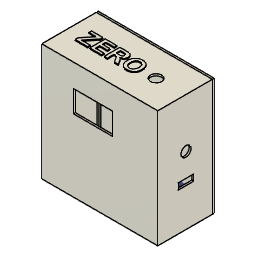
DigitalAngleGauge (Autodesk Fusion 360 design; units mm, degrees)
Autodesk Fusion 360 part; units mm, degrees
note: some values were not read from the file. Set by a fixed rule: which face or edge a step refers to.
sketch "Sketch1" plane through (0, 0, 0) normal (0, 1, 0) x (1, 0, 0)
  line L0 (0, 0) -> (74.4, 0)
  line L1 (74.4, 0) -> (74.4, -35)
  line L2 (74.4, -35) -> (0, -35)
  line L3 (0, -35) -> (0, 0)
  dimension "d15" = 74.4
  dimension "d16" = 35
  constraint horizontal L0
  constraint vertical L1
  constraint horizontal L2
  constraint vertical L3
  constraint coincident L0.start L3.end
  measures "d15" distance of L0.start L0.end
  measures "d16" distance of L0.start L2.end
extrude "Extrude1" add sketch "Sketch1" along normal blind 75 makes body 1
sketch "Sketch2" plane through (0, 0, 0) normal (0, -1, 0) x (1, 0, 0)
  line L0 (74.4, 35) -> (0, 35)
  line L1 (0, 35) -> (0, 0)
  line L2 (0, 0) -> (74.4, 0)
  line L3 (74.4, 0) -> (74.4, 35)
  line L4 (37.2, 0) -> (37.2, 35) construction
  line L5 (0, 35) -> (37.2, 0) construction
  line L6 (37.2, 0) -> (74.4, 35) construction
  circle A0 centre (18.6, 17.5) radius 4.2
  circle A1 centre (55.8, 17.5) radius 4.2
  dimension "d20" = 8.4
  dimension "d21" = 8.4
  constraint midpoint L2 L4.start
  constraint midpoint L0 L4.end
  constraint coincident L0.end L1.start
  constraint coincident L0.start L3.end
  constraint midpoint L5 A0.centre
  constraint midpoint L6 A1.centre
  measures "d20" diameter of A0
  measures "d21" diameter of A1
extrude "Extrude2" cut sketch "Sketch2" against normal blind 2.2 contours A0 | A1 bodies 1
shell "Shell1" thickness 1.2 removed faces 1 at (24.8, 25, 0) on bodies 1
sketch "Sketch3" plane through (0, 75, 0) normal (0, 1, 0) x (-1, 0, 0)
  line L0 (0, 35) -> (-74.4, 35)
  line L1 (-74.4, 35) -> (-74.4, 0)
  line L2 (-74.4, 0) -> (0, 0)
  line L3 (0, 0) -> (0, 35)
  line L4 (-37.2, 35) -> (-74.4, 0) construction
  circle A0 centre (-55.8, 17.5) radius 3.6
  dimension "d29" = 7.2
  constraint midpoint L0 L4.start
  constraint coincident L1.end L2.start
  constraint midpoint L4 A0.centre
  measures "d29" diameter of A0
extrude "Extrude3" cut sketch "Sketch3" against normal up to surface (1.2 mm away) contours A0 bodies 1
sketch "Sketch4" plane through (0, 75, 0) normal (0, 1, 0) x (-1, 0, 0)
  circle A0 centre (-55.8, 17.5) radius 3.6
  line L0 (0, 35) -> (-74.4, 35)
  line L1 (-74.4, 35) -> (-74.4, 0)
  line L2 (-74.4, 0) -> (0, 0)
  line L3 (0, 0) -> (0, 35)
  line L4 (0, 35) -> (-55.8, 35) construction
  line L5 (-55.8, 35) -> (-55.8, 0) construction
  line L6 (-55.8, 0) -> (0, 0) construction
  line L7 (0, 0) -> (0, 35) construction
  dimension "d32" = 10
  text T0 "ZERO" font "Arial" height 10 bold align centre middle in box 55.8 x 35 at (0, 35) x (-1, 0) y (0, -1) spacing 1 kerned
  constraint coincident L0
  constraint coincident L2.end
  constraint coincident A0.centre L5
extrude "Extrude4" add sketch "Sketch4" along normal blind 0.6 text T0 bodies 1
sketch "Sketch5" plane through (1.2, 0, 0) normal (1, 0, 0) x (0, 0, -1)
  line L0 (-33.8, 1.2) -> (0, 1.2)
  line L1 (0, 1.2) -> (0, 73.8)
  line L2 (0, 73.8) -> (-33.8, 73.8)
  line L3 (-33.8, 73.8) -> (-33.8, 1.2)
  line L4 (-33.8, 12.4) -> (0, 12.4) construction
  line L5 (-12.1, 3.4) -> (-22.9, 3.4) construction
  circle A0 centre (-16.9, 12.4) radius 9
  dimension "d36" = 9
  dimension "d37" = 18
  constraint coincident L3 L4.start
  constraint coincident L1 L4.end
  constraint perpendicular L3 L4
  constraint midpoint L4 A0.centre
  measures "d36" distance of L4 L5
  measures "d37" diameter of A0
extrude "Extrude5" add sketch "Sketch5" along normal up to surface (72 mm away) separate body contours A0 makes body 2
sketch "Sketch6" plane through (1.2, 0, 0) normal (1, 0, 0) x (0, 0, -1)
  line L0 (-33.8, 1.2) -> (0, 1.2)
  line L1 (0, 1.2) -> (0, 73.8)
  line L2 (0, 73.8) -> (-33.8, 73.8)
  line L3 (-33.8, 73.8) -> (-33.8, 1.2)
  line L4 (-27.6, 67.1397) -> (-6.2, 67.1397) construction
  line L5 (-6.2, 67.1397) -> (-6.2, 23.6397) construction
  line L6 (-6.2, 23.6397) -> (-27.6, 23.6397) construction
  line L7 (-27.6, 23.6397) -> (-27.6, 67.1397) construction
  line L8 (-6.2, 67.1397) -> (0, 67.1397) construction
  line L9 (-27.6, 67.1397) -> (-33.8, 67.1397) construction
  circle A0 centre (-9.2, 61) radius 1.2
  circle A1 centre (-25.2, 31) radius 1.2
  dimension "d40" = 21.4
  dimension "d41" = 43.5
  dimension "d42" = 3
  dimension "d43" = 19
  dimension "d44" = 2.4
  dimension "d45" = 2.4
  constraint horizontal L4
  constraint vertical L5
  constraint horizontal L6
  constraint vertical L7
  constraint coincident L1 L8.end
  constraint perpendicular L1 L8
  constraint coincident L3 L9.end
  constraint perpendicular L3 L9
  constraint equal L8 L9
  measures "d40" distance of L4.start L4.end
  measures "d41" distance of L4.start L6.end
  measures "d42" distance of L5 A0.centre
  measures "d43" distance of L5 A1.centre
  measures "d44" diameter of A1
  measures "d45" diameter of A0
extrude "Extrude6" add sketch "Sketch6" along normal blind 4 contours A0 | A1 bodies 1
sketch "Sketch7" plane through (73.2, 0, 0) normal (-1, 0, 0) x (0, 0, 1)
  line L0 (0, 1.2) -> (33.8, 1.2)
  line L1 (33.8, 1.2) -> (33.8, 73.8)
  line L2 (33.8, 73.8) -> (0, 73.8)
  line L3 (0, 73.8) -> (0, 1.2)
  line L4 (7.9, 24.4) -> (25.9, 24.4) construction
  line L5 (25.9, 24.4) -> (25.9, 22.4) construction
  line L6 (25.9, 22.4) -> (7.9, 22.4) construction
  line L7 (7.9, 22.4) -> (7.9, 24.4) construction
  line L8 (7.9, 24.4) -> (0, 24.4) construction
  line L9 (25.9, 24.4) -> (33.8, 24.4) construction
  circle A0 centre (16.9, 12.4) radius 9 construction
  line L10 (11.9, 24.4) -> (21.9, 24.4)
  line L11 (21.9, 24.4) -> (21.9, 28.4)
  line L12 (21.9, 28.4) -> (11.9, 28.4)
  line L13 (11.9, 28.4) -> (11.9, 24.4)
  line L14 (21.9, 28.4) -> (25.9, 24.4) construction
  line L15 (11.9, 28.4) -> (7.9, 24.4) construction
  dimension "d48" = 2
  dimension "d49" = 18
  dimension "d50" = 10
  dimension "d51" = 10
  dimension "d52" = 4
  constraint horizontal L4
  constraint vertical L5
  constraint horizontal L6
  constraint vertical L7
  constraint coincident L3 L8.end
  constraint perpendicular L3 L8
  constraint coincident L1 L9.end
  constraint perpendicular L1 L9
  constraint equal L8 L9
  constraint horizontal L10
  constraint vertical L11
  constraint horizontal L12
  constraint vertical L13
  constraint coincident L4 L10.start
  constraint equal L14 L15
  measures "d48" distance of L4.start L6.end
  measures "d49" distance of L4.start L4.end
  measures "d50" distance of L6 A0.centre
  measures "d51" distance of L11.end L12.end
  measures "d52" distance of L10.end L11.end
extrude "Extrude7" cut sketch "Sketch7" against normal up to surface (1.2 mm away) contours L10 L11 L12 L13 bodies 1
sketch "Sketch8" plane through (73.2, 0, 0) normal (-1, 0, 0) x (0, 0, 1)
  line L0 (11.9, 28.4) -> (21.9, 28.4)
  line L1 (21.9, 28.4) -> (21.9, 24.4)
  line L2 (21.9, 24.4) -> (11.9, 24.4)
  line L3 (11.9, 24.4) -> (11.9, 28.4)
  line L4 (0, 1.2) -> (33.8, 1.2)
  line L5 (33.8, 1.2) -> (33.8, 73.8)
  line L6 (33.8, 73.8) -> (0, 73.8)
  line L7 (0, 73.8) -> (0, 1.2)
  circle A0 centre (16.9, 43.4) radius 3.25
  line L8 (16.9, 43.4) -> (0, 43.4) construction
  line L9 (16.9, 43.4) -> (33.8, 43.4) construction
  dimension "d55" = 15
  dimension "d56" = 6.5
  constraint coincident A0.centre L8.start
  constraint coincident L7 L8.end
  constraint perpendicular L7 L8
  constraint coincident L5 L9.end
  constraint perpendicular L5 L9
  constraint equal L8 L9
  measures "d55" distance of L0 A0.centre
  measures "d56" diameter of A0
extrude "Extrude8" cut sketch "Sketch8" against normal up to surface (1.2 mm away) contours A0 bodies 1
sketch "Sketch9" plane through (0, 0, 33.8) normal (0, 0, -1) x (-1, 0, 0)
  line L0 (-73.2, 1.2) -> (-1.2, 1.2)
  line L1 (-1.2, 1.2) -> (-1.2, 73.8)
  line L2 (-1.2, 73.8) -> (-73.2, 73.8)
  line L3 (-73.2, 73.8) -> (-73.2, 1.2)
  line L4 (-1.2, 68.2) -> (-14.2, 68.2) construction
  line L5 (-14.2, 68.2) -> (-14.2, 25.2) construction
  line L6 (-14.2, 25.2) -> (-1.2, 25.2) construction
  line L7 (-1.2, 25.2) -> (-1.2, 68.2) construction
  line L8 (-5.2, 62.2) -> (-5.2, 59.8) construction
  line L9 (-1.2, 59.8) -> (-1.2, 62.2) construction
  line L10 (-73.2, 73.8) -> (-50.2, 73.8) construction
  line L11 (-50.2, 73.8) -> (-50.2, 21.4) construction
  line L12 (-50.2, 21.4) -> (-73.2, 21.4) construction
  line L13 (-73.2, 21.4) -> (-73.2, 73.8) construction
  line L14 (-1.2, 21.4) -> (-1.2, 3.4) construction
  line L15 (-73.2, 21.4) -> (-73.2, 3.4) construction
  line L16 (-46.4, 65.8) -> (-19.2, 65.8) construction
  line L17 (-19.2, 65.8) -> (-19.2, 37.8) construction
  line L18 (-19.2, 37.8) -> (-46.4, 37.8) construction
  line L19 (-46.4, 37.8) -> (-46.4, 65.8) construction
  line L20 (-45.3, 60.3) -> (-20.3, 60.3)
  line L21 (-20.3, 60.3) -> (-20.3, 46.3)
  line L22 (-20.3, 46.3) -> (-45.3, 46.3)
  line L23 (-45.3, 46.3) -> (-45.3, 60.3)
  line L24 (-45.3, 53.3) -> (-46.4, 53.3) construction
  line L25 (-20.3, 53.3) -> (-19.2, 53.3) construction
  line L26 (-46.4, 37.8) -> (-42.6, 37.8)
  line L27 (-42.6, 37.8) -> (-42.6, 36.6)
  line L28 (-42.6, 36.6) -> (-47.6, 36.6)
  line L29 (-47.6, 36.6) -> (-47.6, 41.6)
  line L30 (-47.6, 41.6) -> (-46.4, 41.6)
  line L31 (-46.4, 37.8) -> (-46.4, 41.6)
  line L32 (-46.4, 37.8) -> (-19.2, 65.8) construction
  line L33 (-19.2, 37.8) -> (-46.4, 65.8) construction
  line L34 (-19.2, 37.8) -> (-23, 37.8)
  line L35 (-23, 37.8) -> (-23, 36.6)
  line L36 (-23, 36.6) -> (-18, 36.6)
  line L37 (-18, 36.6) -> (-18, 41.6)
  line L38 (-18, 41.6) -> (-19.2, 41.6)
  line L39 (-19.2, 37.8) -> (-19.2, 41.6)
  line L40 (-19.2, 62) -> (-18, 62)
  line L41 (-18, 62) -> (-18, 67)
  line L42 (-18, 67) -> (-23, 67)
  line L43 (-23, 67) -> (-23, 65.8)
  line L44 (-19.2, 65.8) -> (-23, 65.8)
  line L45 (-19.2, 65.8) -> (-19.2, 62)
  line L46 (-46.4, 65.8) -> (-42.6, 65.8)
  line L47 (-42.6, 65.8) -> (-42.6, 67)
  line L48 (-42.6, 67) -> (-47.6, 67)
  line L49 (-47.6, 67) -> (-47.6, 62)
  line L50 (-47.6, 62) -> (-46.4, 62)
  line L51 (-46.4, 65.8) -> (-46.4, 62)
  dimension "d59" = 13
  dimension "d60" = 43
  dimension "d61" = 6
  dimension "d62" = 23
  dimension "d63" = 27.2
  dimension "d64" = 28
  dimension "d65" = 5
  dimension "d66" = 8
  dimension "d67" = 5.5
  dimension "d68" = 25
  dimension "d69" = 14
  dimension "d70" = 1.2
  dimension "d71" = 1.2
  dimension "d72" = 5
  dimension "d73" = 5
  dimension "d74" = 1.2
  dimension "d75" = 1.2
  dimension "d76" = 1.2
  dimension "d77" = 1.2
  dimension "d78" = 5
  dimension "d79" = 5
  dimension "d80" = 5
  dimension "d81" = 5
  dimension "d82" = 1.2
  dimension "d83" = 1.2
  dimension "d84" = 5
  dimension "d85" = 5
  constraint horizontal L4
  constraint vertical L5
  constraint horizontal L6
  constraint vertical L7
  constraint coincident L1 L4.start
  constraint horizontal L10
  constraint vertical L11
  constraint horizontal L12
  constraint vertical L13
  constraint coincident L3 L2.end
  constraint collinear L2 L10
  constraint coincident L12 L13.start
  constraint horizontal L16
  constraint vertical L17
  constraint horizontal L18
  constraint vertical L19
  constraint horizontal L20
  constraint vertical L21
  constraint horizontal L22
  constraint vertical L23
  constraint midpoint L23 L24.start
  constraint coincident L19 L24.end
  constraint perpendicular L19 L24
  constraint midpoint L21 L25.start
  constraint coincident L17 L25.end
  constraint perpendicular L17 L25
  constraint equal L24 L25
  constraint coincident L18 L26.end
  constraint perpendicular L19 L26
  constraint perpendicular L26 L27
  constraint perpendicular L27 L28
  constraint perpendicular L28 L29
  constraint coincident L19 L30.end
  constraint perpendicular L19 L30
  constraint coincident L18 L34.end
  constraint perpendicular L17 L34
  constraint perpendicular L18 L35
  constraint perpendicular L35 L36
  constraint perpendicular L36 L37
  constraint coincident L17 L38.end
  constraint perpendicular L17 L38
  constraint coincident L17 L40.start
  constraint perpendicular L17 L40
  constraint perpendicular L40 L41
  constraint perpendicular L17 L42
  constraint coincident L16 L43.end
  constraint perpendicular L16 L43
  constraint coincident L16 L46.end
  constraint perpendicular L19 L46
  constraint perpendicular L46 L47
  constraint perpendicular L47 L48
  constraint perpendicular L46 L49
  constraint coincident L19 L50.end
  constraint perpendicular L19 L50
  measures "d59" distance of L4.start L4.end
  measures "d60" distance of L4.end L5.end
  measures "d61" distance of L4 L8.start
  measures "d62" distance of L2.end L10.end
  measures "d63" distance of L16.start L16.end
  measures "d64" distance of L16.start L18.end
  measures "d65" distance of L5 L17
  measures "d66" distance of L2 L16
  measures "d67" distance of L16 L20
  measures "d68" distance of L20.start L20.end
  measures "d69" distance of L20.start L22.end
  measures "d70" distance of L18 L28
  measures "d71" distance of L19 L29
  measures "d72" distance of L28 L30
  measures "d73" distance of L27 L29
  measures "d74" distance of L40.start L40.end
  measures "d75" distance of L42.end L43.end
  measures "d76" distance of L37.end L38.end
  measures "d77" distance of L34.end L35.end
  measures "d78" distance of L35.end L36.end
  measures "d79" distance of L36.end L37.end
  measures "d80" distance of L40.end L41.end
  measures "d81" distance of L41.end L42.end
  measures "d82" distance of L49.end L50.end
  measures "d83" distance of L46.end L47.end
  measures "d84" distance of L47.end L48.end
  measures "d85" distance of L48.end L49.end
extrude "Extrude9" cut sketch "Sketch9" against normal up to surface (1.2 mm away) contours L20 L21 L22 L23 bodies 1
extrude "Extrude10" add sketch "Sketch9" along normal blind 4 contours L26 L27 L28 L29 L30 L31 | L34 L35 L36 L37 L38 L39 | L40 L41 L42 L43 L44 L45 | L46 L47 L48 L49 L50 L51 bodies 1
sketch "Sketch10" plane through (0, 0, 0) normal (0, 0, -1) x (-1, 0, 0)
  line L0 (-73.2, 1.2) -> (-73.2, 73.8)
  line L1 (-73.2, 73.8) -> (-1.2, 73.8)
  line L2 (-1.2, 73.8) -> (-1.2, 1.2)
  line L3 (-1.2, 1.2) -> (-73.2, 1.2)
  line L4 (-74.4, 0) -> (0, 0)
  line L5 (0, 0) -> (0, 75)
  line L6 (0, 75) -> (-74.4, 75)
  line L7 (-74.4, 75) -> (-74.4, 0)
  line L8 (-73.2, 1.2) -> (-65.2, 1.2)
  line L9 (-65.2, 1.2) -> (-65.2, 9.2)
  line L10 (-65.2, 9.2) -> (-73.2, 9.2)
  line L11 (-73.2, 9.2) -> (-73.2, 1.2)
  line L12 (-1.2, 1.2) -> (-9.2, 1.2)
  line L13 (-9.2, 1.2) -> (-9.2, 9.2)
  line L14 (-9.2, 9.2) -> (-1.2, 9.2)
  line L15 (-1.2, 9.2) -> (-1.2, 1.2)
  line L16 (-1.2, 73.8) -> (-9.2, 73.8)
  line L17 (-9.2, 73.8) -> (-9.2, 65.8)
  line L18 (-9.2, 65.8) -> (-1.2, 65.8)
  line L19 (-1.2, 65.8) -> (-1.2, 73.8)
  line L20 (-73.2, 73.8) -> (-65.2, 73.8)
  line L21 (-65.2, 73.8) -> (-65.2, 65.8)
  line L22 (-65.2, 65.8) -> (-73.2, 65.8)
  line L23 (-73.2, 65.8) -> (-73.2, 73.8)
  dimension "d93" = 8
  dimension "d94" = 8
  dimension "d95" = 8
  dimension "d96" = 8
  dimension "d97" = 8
  dimension "d98" = 8
  dimension "d99" = 8
  dimension "d100" = 8
  constraint horizontal L8
  constraint vertical L9
  constraint horizontal L10
  constraint vertical L11
  constraint coincident L0.start L3.end
  constraint horizontal L12
  constraint vertical L13
  constraint horizontal L14
  constraint vertical L15
  constraint coincident L2.end L3.start
  constraint horizontal L16
  constraint vertical L17
  constraint horizontal L18
  constraint vertical L19
  constraint coincident L1.end L2.start
  constraint horizontal L20
  constraint vertical L21
  constraint horizontal L22
  constraint vertical L23
  constraint coincident L0.end L1.start
  measures "d93" distance of L0.start L8.end
  measures "d94" distance of L0.start L10.end
  measures "d95" distance of L2.end L14.end
  measures "d96" distance of L2.end L12.end
  measures "d97" distance of L1.end L16.end
  measures "d98" distance of L1.end L18.end
  measures "d99" distance of L0.end L20.end
  measures "d100" distance of L0.end L22.end
extrude "Extrude11" add sketch "Sketch10" against normal blind 15 contours L0 L3 L8 L9 L10 L11 | L0 L1 L20 L21 L22 L23 | L2 L3 L12 L13 L14 L15 | L1 L2 L16 L17 L18 L19 bodies 1
sketch "Sketch11" plane through (0, 0, 0) normal (0, 0, -1) x (-1, 0, 0)
  line L0 (-73.2, 9.2) -> (-73.2, 65.8)
  line L1 (-73.2, 65.8) -> (-65.2, 65.8)
  line L2 (-65.2, 65.8) -> (-65.2, 73.8)
  line L3 (-65.2, 73.8) -> (-9.2, 73.8)
  line L4 (-9.2, 73.8) -> (-9.2, 65.8)
  line L5 (-9.2, 65.8) -> (-1.2, 65.8)
  line L6 (-1.2, 65.8) -> (-1.2, 9.2)
  line L7 (-1.2, 9.2) -> (-9.2, 9.2)
  line L8 (-9.2, 9.2) -> (-9.2, 1.2)
  line L9 (-9.2, 1.2) -> (-65.2, 1.2)
  line L10 (-65.2, 1.2) -> (-65.2, 9.2)
  line L11 (-65.2, 9.2) -> (-73.2, 9.2)
  line L12 (-74.4, 0) -> (0, 0)
  line L13 (0, 0) -> (0, 75)
  line L14 (0, 75) -> (-74.4, 75)
  line L15 (-74.4, 75) -> (-74.4, 0)
  line L16 (-73.2, 65.8) -> (-65.2, 73.8) construction
  line L17 (-9.2, 73.8) -> (-1.2, 65.8) construction
  line L18 (-1.2, 9.2) -> (-9.2, 1.2) construction
  line L19 (-65.2, 1.2) -> (-73.2, 9.2) construction
  circle A0 centre (-69.2, 5.2) radius 1.4
  circle A1 centre (-69.2, 69.8) radius 1.4
  circle A2 centre (-5.2, 69.8) radius 1.4
  circle A3 centre (-5.2, 5.2) radius 1.4
  dimension "d103" = 2.8
  dimension "d104" = 2.8
  dimension "d105" = 2.8
  dimension "d106" = 2.8
  constraint coincident L0.end L1.start
  constraint coincident L2.end L3.start
  constraint coincident L3.end L4.start
  constraint coincident L5.end L6.start
  constraint coincident L6.end L7.start
  constraint coincident L8.end L9.start
  constraint coincident L9.end L10.start
  constraint coincident L0.start L11.end
  constraint midpoint L19 A0.centre
  constraint midpoint L16 A1.centre
  constraint midpoint L17 A2.centre
  constraint midpoint L18 A3.centre
  measures "d103" diameter of A0
  measures "d104" diameter of A1
  measures "d105" diameter of A2
  measures "d106" diameter of A3
extrude "Extrude12" cut sketch "Sketch11" against normal blind 13.5 contours A0 | A1 | A2 | A3 bodies 1 2
sketch "Sketch12" plane through (0, 0, 0) normal (0, 0, -1) x (-1, 0, 0)
  circle A0 centre (-69.2, 5.2) radius 1.4
  circle A1 centre (-69.2, 69.8) radius 1.4
  circle A2 centre (-5.2, 5.2) radius 1.4
  circle A3 centre (-5.2, 69.8) radius 1.4
  line L0 (-73.2, 9.2) -> (-73.2, 65.8)
  line L1 (-73.2, 65.8) -> (-65.2, 65.8)
  line L2 (-65.2, 65.8) -> (-65.2, 73.8)
  line L3 (-65.2, 73.8) -> (-9.2, 73.8)
  line L4 (-9.2, 73.8) -> (-9.2, 65.8)
  line L5 (-9.2, 65.8) -> (-1.2, 65.8)
  line L6 (-1.2, 65.8) -> (-1.2, 9.2)
  line L7 (-1.2, 9.2) -> (-9.2, 9.2)
  line L8 (-9.2, 9.2) -> (-9.2, 1.2)
  line L9 (-9.2, 1.2) -> (-65.2, 1.2)
  line L10 (-65.2, 1.2) -> (-65.2, 9.2)
  line L11 (-65.2, 9.2) -> (-73.2, 9.2)
  line L12 (-74.4, 0) -> (0, 0)
  line L13 (0, 0) -> (0, 75)
  line L14 (0, 75) -> (-74.4, 75)
  line L15 (-74.4, 75) -> (-74.4, 0)
  line L16 (-74.4, 75) -> (0, 75)
  line L17 (0, 75) -> (0, 0)
  line L18 (0, 0) -> (-74.4, 0)
  line L19 (-74.4, 0) -> (-74.4, 75)
  constraint horizontal L16
  constraint vertical L17
  constraint horizontal L18
  constraint vertical L19
  constraint coincident L12.end L13.start
  constraint coincident L14.end L15.start
extrude "Extrude13" add sketch "Sketch12" along normal blind 1.2 separate body contours L0 L1 L2 L3 L4 L5 L6 L7 L8 L9 L10 L11 | L12 L13 L14 L15 L16 L17 L18 L19 makes body 3
chamfer "Chamfer1" distance 0.6 angle 45 4 edges at (70.5053, 70.3063, -1.2) (70.5053, 5.7063, -1.2) (6.5053, 5.7063, -1.2) (6.5053, 70.3063, -1.2) on bodies 3
sketch "Sketch13" plane through (0, 0, 0) normal (0, 0, 1) x (1, 0, 0)
  circle A0 centre (5.2, 5.2) radius 1.4
  circle A1 centre (69.2, 69.8) radius 1.4
  circle A2 centre (5.2, 69.8) radius 1.4
  circle A3 centre (69.2, 5.2) radius 1.4
  line L0 (0, 0) -> (74.4, 0)
  line L1 (74.4, 0) -> (74.4, 75)
  line L2 (74.4, 75) -> (0, 75)
  line L3 (0, 75) -> (0, 0)
  circle A4 centre (69.2, 5.2) radius 1.4
  circle A5 centre (69.2, 69.8) radius 1.4
  circle A6 centre (5.2, 5.2) radius 1.4
  circle A7 centre (5.2, 69.8) radius 1.4
  line L4 (73.2, 9.2) -> (73.2, 65.8)
  line L5 (73.2, 65.8) -> (65.2, 65.8)
  line L6 (65.2, 65.8) -> (65.2, 73.8)
  line L7 (65.2, 73.8) -> (9.2, 73.8)
  line L8 (9.2, 73.8) -> (9.2, 65.8)
  line L9 (9.2, 65.8) -> (1.2, 65.8)
  line L10 (1.2, 65.8) -> (1.2, 9.2)
  line L11 (1.2, 9.2) -> (9.2, 9.2)
  line L12 (9.2, 9.2) -> (9.2, 1.2)
  line L13 (9.2, 1.2) -> (65.2, 1.2)
  line L14 (65.2, 1.2) -> (65.2, 9.2)
  line L15 (65.2, 9.2) -> (73.2, 9.2)
  line L16 (74.4, 0) -> (0, 0)
  line L17 (0, 0) -> (0, 75)
  line L18 (0, 75) -> (74.4, 75)
  line L19 (74.4, 75) -> (74.4, 0)
  line L20 (1.7, 9.2) -> (1.7, 65.8)
  line L21 (9.2, 73.3) -> (65.2, 73.3)
  line L22 (72.7, 65.8) -> (72.7, 9.2)
  line L23 (65.2, 1.7) -> (9.2, 1.7)
  line L24 (2.9, 65.8) -> (2.9, 9.2)
  line L25 (9.2, 2.9) -> (65.2, 2.9)
  line L26 (71.5, 9.2) -> (71.5, 65.8)
  line L27 (65.2, 72.1) -> (9.2, 72.1)
  line L28 (9.7, 73.3) -> (9.7, 72.1)
  line L29 (1.7, 65.3) -> (2.9, 65.3)
  line L30 (64.7, 73.3) -> (64.7, 72.1)
  line L31 (71.5, 65.3) -> (72.7, 65.3)
  line L32 (64.7, 2.9) -> (64.7, 1.7)
  line L33 (71.5, 9.7) -> (72.7, 9.7)
  line L34 (9.7, 2.9) -> (9.7, 1.7)
  line L35 (1.7, 9.7) -> (2.9, 9.7)
  dimension "d115" = 0.5
  dimension "d116" = 0.5
  dimension "d117" = 0.5
  dimension "d118" = 0.5
  dimension "d119" = 1.2
  dimension "d120" = 1.2
  dimension "d121" = 1.2
  dimension "d122" = 1.2
  dimension "d123" = 0.5
  dimension "d124" = 0.5
  dimension "d125" = 0.5
  dimension "d126" = 0.5
  dimension "d127" = 0.5
  dimension "d128" = 0.5
  dimension "d129" = 0.5
  dimension "d130" = 0.5
  constraint coincident L11 L20.start
  constraint coincident L9 L20.end
  constraint perpendicular L9 L20
  constraint coincident L8 L21.start
  constraint coincident L6 L21.end
  constraint perpendicular L6 L21
  constraint coincident L5 L22.start
  constraint coincident L15 L22.end
  constraint perpendicular L15 L22
  constraint coincident L14 L23.start
  constraint coincident L12 L23.end
  constraint perpendicular L12 L23
  constraint coincident L9 L24.start
  constraint coincident L11 L24.end
  constraint perpendicular L11 L24
  constraint coincident L12 L25.start
  constraint coincident L14 L25.end
  constraint perpendicular L14 L25
  constraint coincident L15 L26.start
  constraint coincident L5 L26.end
  constraint perpendicular L5 L26
  constraint coincident L6 L27.start
  constraint coincident L8 L27.end
  constraint perpendicular L8 L27
  constraint coincident L21 L28.start
  constraint coincident L27 L28.end
  constraint perpendicular L27 L28
  constraint coincident L20 L29.start
  constraint coincident L24 L29.end
  constraint perpendicular L24 L29
  constraint coincident L21 L30.start
  constraint coincident L27 L30.end
  constraint perpendicular L27 L30
  constraint coincident L26 L31.start
  constraint coincident L22 L31.end
  constraint perpendicular L22 L31
  constraint coincident L25 L32.start
  constraint coincident L23 L32.end
  constraint perpendicular L23 L32
  constraint coincident L26 L33.start
  constraint coincident L22 L33.end
  constraint perpendicular L22 L33
  constraint coincident L25 L34.start
  constraint coincident L23 L34.end
  constraint perpendicular L23 L34
  constraint coincident L20 L35.start
  constraint coincident L24 L35.end
  constraint perpendicular L24 L35
  measures "d115" distance of L13 L23
  measures "d116" distance of L4 L22
  measures "d117" distance of L7 L21
  measures "d118" distance of L10 L20
  measures "d119" distance of L21 L27
  measures "d120" distance of L20 L24
  measures "d121" distance of L22 L26
  measures "d122" distance of L23 L25
  measures "d123" distance of L9 L29
  measures "d124" distance of L8 L28
  measures "d125" distance of L5 L31
  measures "d126" distance of L6 L30
  measures "d127" distance of L15 L33
  measures "d128" distance of L14 L32
  measures "d129" distance of L12 L34.start
  measures "d130" distance of L11 L35
extrude "Extrude14" add sketch "Sketch13" along normal blind 1.2 contours L22 L26 L31 L33 | L23 L25 L32 L34 | L21 L27 L28 L30 | L20 L24 L29 L35 bodies 3
move_face "OffsetFaces1" offset -0.4 4 faces at (68.6242, 71.0761, -0.4) (3.8844, 69.3212, -0.4) (69.0259, 6.5891, -0.4) (3.8017, 5.1302, -0.4) on bodies 3
chamfer "Chamfer2" distance 8 angle 45 4 edges at (5.2, 9.2, 15) (69.2, 9.2, 15) (69.2, 65.8, 15) (5.2, 65.8, 15) on bodies 1
equation "OnSwitchHoleDiameter = 6.5 mm"
equation "ZeroButtonHoleDiameter = 7.2 mm"
equation "USBCWidth = 10 mm"
equation "USBCHeight = 4 mm"
equation "OLEDWidth = 27.2 mm"
equation "OLEDHeight = 28 mm"
equation "DisplayHeight = 14 mm"
equation "DisplayWidth = 25 mm"
equation "DisplayTopOffset = 5.5 mm"
equation "USBMiniWidth = 8 mm"
equation "USBMiniHeight = 4.5 mm"
equation "CaseWidth = BatteryLength + 2 * CaseWallThickness"
equation "CaseDepth = 35 mm"
equation "CaseHeight = 75 mm"
equation "d15 = CaseWidth"
equation "d16 = CaseDepth"
equation "d17 = CaseHeight"
equation "MagnetHoleSize = 8.4 mm"
equation "d20 = MagnetHoleSize"
equation "d21 = MagnetHoleSize"
equation "MagnetHoleDepth = 2.2 mm"
equation "d23 = -MagnetHoleDepth"
equation "CaseWallThickness = ( 0.6 * 2 ) * 1 mm"
equation "d26 = CaseWallThickness"
equation "BatteryDiameter = 18 mm"
equation "BatteryLength = 72 mm"
equation "d29 = ZeroButtonHoleDiameter"
equation "TextDepth = ( 0.2 * 3 ) * 1 mm"
equation "d34 = TextDepth"
equation "d36 = BatteryDiameter / 2"
equation "d37 = BatteryDiameter"
equation "d50 = BatteryDiameter / 2 + 1 mm"
equation "d51 = USBCWidth"
equation "d52 = USBCHeight"
equation "d56 = OnSwitchHoleDiameter"
equation "d63 = OLEDWidth"
equation "d64 = OLEDHeight"
equation "d67 = DisplayTopOffset"
equation "d68 = DisplayWidth"
equation "d69 = DisplayHeight"
equation "d70 = CaseWallThickness"
equation "d71 = CaseWallThickness"
equation "d74 = CaseWallThickness"
equation "d75 = CaseWallThickness"
equation "d76 = CaseWallThickness"
equation "d77 = CaseWallThickness"
equation "d82 = CaseWallThickness"
equation "d83 = CaseWallThickness"
equation "LidHoleSize = 2.8 mm"
equation "LidStandThickness = 8 mm"
equation "LidStandHeight = 15 mm"
equation "d93 = LidStandThickness"
equation "d94 = LidStandThickness"
equation "d95 = LidStandThickness"
equation "d96 = LidStandThickness"
equation "d97 = LidStandThickness"
equation "d98 = LidStandThickness"
equation "d99 = LidStandThickness"
equation "d100 = LidStandThickness"
equation "d101 = -LidStandHeight"
equation "d103 = LidHoleSize"
equation "d104 = LidHoleSize"
equation "d105 = LidHoleSize"
equation "d106 = LidHoleSize"
equation "d107 = -LidStandHeight * 0.9"
equation "LidThickness = CaseWallThickness"
equation "d110 = LidThickness"
equation "d112 = LidThickness / 2"
equation "LidRibOffset = 0.5 mm"
equation "LidRibThickness = CaseWallThickness"
equation "d115 = LidRibOffset"
equation "d116 = LidRibOffset"
equation "d117 = LidRibOffset"
equation "d118 = LidRibOffset"
equation "d119 = LidRibThickness"
equation "d120 = LidRibThickness"
equation "d121 = LidRibThickness"
equation "d122 = LidRibThickness"
equation "d123 = LidRibOffset"
equation "d124 = LidRibOffset"
equation "d125 = LidRibOffset"
equation "d126 = LidRibOffset"
equation "d127 = LidRibOffset"
equation "d128 = LidRibOffset"
equation "d129 = LidRibOffset"
equation "d130 = LidRibOffset"
equation "d131 = LidRibThickness"
equation "d133 = -LidHoleEnlargement"
equation "LidHoleEnlargement = 0.4 mm"
equation "d135 = LidStandThickness"
named bodies: "Body", "Battery", "Lid"
